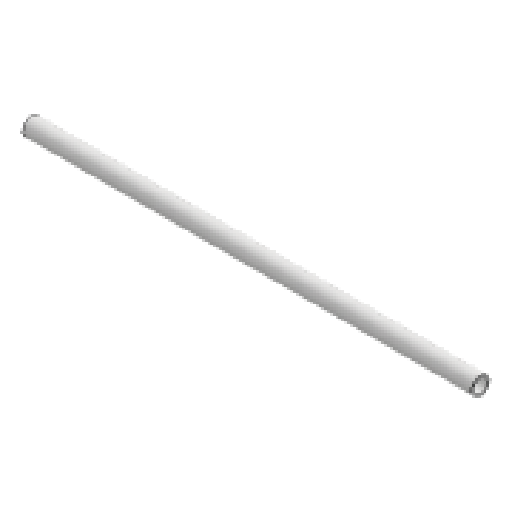
# Autodesk Inventor part: CarbonHorizontalSlideCrossbar
Saved by Autodesk Inventor 2023 (Build 270158000, 158)
## iProperties
Created: 2022-10-31
Part Number: CarbonHorizontalSlideCrossbar
Material: CFRP
Document SubType Name: Modeling
Designer: deli
Density: 1.43 g/cm^3
Appearance: Carbon Fiber
Author: deli
Autodesk Inventor part; units mm, degrees
ref_plane "YZ Plane" through (0, 0, 0) normal (1, 0, 0) x (0, 1, 0)
ref_plane "XZ Plane" through (0, 0, 0) normal (0, 1, 0) x (-1, 0, 0)
ref_plane "XY Plane" through (0, 0, 0) normal (0, 0, 1) x (1, 0, 0)
sketch "Sketch1" plane through (0, 0, 0) normal (1, 0, 0) x (0, 1, 0)
  circle A0 centre (23.3286, -15.6674) radius 3
  circle A1 centre (23.3286, -15.6674) radius 4
  point P0 (0, 0)
  dimension "d0" = 6
  dimension "d1" = 8
  constraints: 2 centre point, 1 coincident
  measures "d0" diameter of A0
  measures "d1" diameter of A1
extrude "Extrusion1" add sketch "Sketch1" along normal blind 200
body "Solid1"
